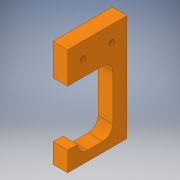
# Autodesk Inventor part: hook
Saved by Autodesk Inventor 2019 (Build 230136000, 136)
## iProperties
Created: 2018-09-20
Part Number: hook
Material: Generic
Document SubType Name: Modeling
Designer: User
Density: 1 g/cm^3
Appearance: Orange
Author: User
Autodesk Inventor part; units mm, degrees
ref_plane "YZ Plane" through (0, 0, 0) normal (1, 0, 0) x (0, 1, 0)
ref_plane "XZ Plane" through (0, 0, 0) normal (0, 1, 0) x (-1, 0, 0)
ref_plane "XY Plane" through (0, 0, 0) normal (0, 0, 1) x (1, 0, 0)
sketch "Sketch1" plane through (0, 0, 0) normal (1, 0, 0) x (0, 1, 0)
  line L0 (0, 0) -> (0, -38.1)
  line L1 (0, -38.1) -> (68.58, -38.1)
  line L2 (68.58, -38.1) -> (68.58, -28.956)
  line L3 (68.58, -28.956) -> (6.35, -28.956)
  line L4 (0, 0) -> (12.7, 0)
  line L5 (12.7, 0) -> (12.7, -6.35)
  line L6 (12.7, -6.35) -> (6.35, -6.35)
  line L7 (0, 0) -> (6.35, 0)
  line L8 (6.35, -6.35) -> (6.35, -28.956)
  line L9 (68.58, -38.1) -> (48.26, -38.1)
  line L10 (48.26, -38.1) -> (48.26, 0)
  line L11 (48.26, 0) -> (68.58, 0)
  line L12 (68.58, 0) -> (68.58, -38.1)
  dimension "d0" = 38.1
  dimension "d1" = 68.58
  dimension "d2" = 9.144
  dimension "d3" = 6.35
  dimension "d4" = 12.7
  dimension "d5" = 6.35
  dimension "d6" = 6.35
  dimension "d10" = 20.32
  dimension "d11" = 38.1
  constraints: 26 end point, 6 perpendicular, 2 horizontal, 2 parallel, 1 midpoint, 1 vertical
  measures "d0" distance of L0.start L0.end
  measures "d1" distance of L0.end L1.end
  measures "d2" distance of L1.end L2.end
  measures "d3" distance of L4.end L5.end
  measures "d4" distance between parallel lines of L0 L5
  measures "d5" distance of L0.start L7.end
  measures "d6" distance between parallel lines of L0 L8
  measures "d10" distance of L10.end L11.end
  measures "d11" distance of L9.end L10.end
extrude "Extrusion2" add sketch "Sketch1" along normal blind 9.398
sketch "Sketch2" plane through (9.398, 0, 0) normal (1, 0, 0) x (0, 0, -1)
  line L0 (28.956, 48.26) -> (28.956, 6.35) projected
  line L1 (28.956, 6.35) -> (6.35, 6.35) projected
  line L2 (6.35, 6.35) -> (6.35, 12.7) projected
  line L3 (6.35, 12.7) -> (0, 12.7) projected
  line L4 (0, 12.7) -> (0, 0) projected
  line L5 (0, 0) -> (38.1, 0) projected
  line L6 (38.1, 0) -> (38.1, 68.58) projected
  line L7 (38.1, 68.58) -> (0, 68.58) projected
  line L8 (0, 68.58) -> (0, 48.26) projected
  line L9 (0, 48.26) -> (28.956, 48.26) projected
  point P0 (28.2575, 58.42)
  point P1 (9.8425, 58.42)
  dimension "d14" = 18.415
  dimension "d15" = 38.1
  dimension "d16" = 9.8425
  dimension "d17" = 20.32
  dimension "d18" = 10.16
  dimension "d19" = 10.16
  measures "d14" distance of point (28.257, 58.42) point (9.842, 58.42)
  measures "d15" distance of L6.end L7.end
  measures "d16" distance from line of L6 point (28.257, 58.42)
  measures "d17" distance of L7.end L8.end
  measures "d18" distance from line of L7 point (9.842, 58.42)
  measures "d19" distance from line of L7 point (28.257, 58.42)
hole "Hole1" at (9.398, 58.42, -28.2575) at (9.398, 58.42, -9.8425) direction (-1, 0, 0) diameter 3.556 depth 10.9728 tip angle 118
fillet "Fillet2" radius 6.35 3 edges at (4.699, 6.35, -6.35) (4.699, 6.35, -28.956) (4.699, 48.26, -28.956)
equation "\"d16\" = -0.5 * d14 + 0.5 * d15"
equation "\"d18\" = 0.5 * d17"
equation "\"d19\" = d18"
body "Solid2"
